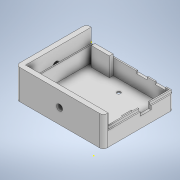
# Autodesk Inventor part: Shell 5 top
Saved by Autodesk Inventor 2022 (Build 260153000, 153)
## iProperties
Created: 2021-10-12
Part Number: Shell 5 top
Material: Generic
Document SubType Name: Modeling
Designer: Elisabeth
Density: 1 g/cm^3
Appearance: Default
Mass: 24.7843 g
Surface Area: 176.522 cm^2
Volume: 24.7843 cm^3
Author: Elisabeth
Autodesk Inventor part; units mm, degrees
ref_plane "YZ Plane" through (0, 0, 0) normal (1, 0, 0) x (0, 1, 0)
ref_plane "XZ Plane" through (0, 0, 0) normal (0, 1, 0) x (-1, 0, 0)
ref_plane "XY Plane" through (0, 0, 0) normal (0, 0, 1) x (1, 0, 0)
sketch "Sketch1" plane through (0, 0, 0) normal (0, 1, 0) x (-1, 0, 0)
  point P0 (0, 0)
sketch "Sketch2" plane through (0, 0, 0) normal (0, 1, 0) x (-1, 0, 0)
  line L0 (68, -12) -> (68, -66)
  line L1 (68, -66) -> (0, -66)
  line L2 (0, -66) -> (0, -12)
  line L3 (68, -12) -> (0, -12)
  point P0 (0, 0)
  dimension "d0" = 68
  dimension "d138" = 54
  constraints: 8 end point, 1 parallel, 1 perpendicular
  measures "d0" distance of L0.end L1.end
  measures "d138" distance between parallel lines of L3 L1
extrude "Extrusion1" add sketch "Sketch2" along normal blind 14
sketch "Sketch3" plane through (0, 14, 0) normal (0, 1, 0) x (1, 0, 0)
  point P0 (-68, 66)
sketch "Sketch4" plane through (0, 14, 0) normal (0, 1, 0) x (1, 0, 0)
  line L0 (0, 66) -> (-68, 66) projected
  line L1 (-30.4814, 66) -> (-28.4814, 66)
  line L2 (-28.4814, 66) -> (-28.4814, 64)
  line L3 (-68, 66) -> (-68, 12) projected
  line L4 (-68, 37.8423) -> (-68, 39.8423)
  line L5 (-68, 39.8423) -> (-66, 39.8423)
  line L6 (0, 38.8423) -> (0, 36.8423)
  line L7 (0, 36.8423) -> (-2, 36.8423)
  line L8 (-66, 64) -> (-2, 64)
  line L9 (-2, 64) -> (-2, 14)
  line L10 (-2, 14) -> (-66, 14)
  line L11 (-66, 14) -> (-66, 64)
  dimension "d5" = 2
  dimension "d6" = 2
  dimension "d7" = 2
  dimension "d11" = 2
  dimension "d75" = 2
  dimension "d132" = 50
  dimension "d133" = 64
  constraints: 20 end point, 4 perpendicular, 4 point on line, 2 parallel, 1 horizontal
  measures "d5" distance of L1.start L1.end
  measures "d6" distance of L1.end L2.end
  measures "d7" distance of L4.start L4.end
  measures "d11" distance of L6.start L6.end
  measures "d75" distance between parallel lines of L0 L8
  measures "d132" distance between parallel lines of L8 L10
  measures "d133" distance of L8.start L8.end
extrude "Extrusion2" cut sketch "Sketch4" against normal blind 13 contours L8 L9 L10 L11
sketch "Sketch7" plane through (0, 14, 0) normal (0, 1, 0) x (1, 0, 0)
  line L0 (-68, 66) -> (-67, 66)
  line L1 (-68, 66) -> (-6, 66)
  line L2 (-68, 65) -> (-68, 66)
  line L3 (0, 66) -> (-7, 66)
  line L4 (-67, 65) -> (-1, 65)
  line L5 (0, 66) -> (-68, 66) projected
  line L6 (-68, 66) -> (0, 66)
  line L7 (0, 12) -> (0, 66) projected
  line L8 (0, 12) -> (-1, 12)
  line L9 (-1, 66) -> (0, 66)
  line L10 (0, 66) -> (0, 12)
  line L11 (0, 12) -> (-1, 12)
  line L12 (-68, 12) -> (0, 12) projected
  line L13 (-1, 65) -> (-1, 12)
  line L14 (0, 12) -> (-1, 12)
  line L15 (-67, 65) -> (-67, 12)
  line L16 (-68, 66) -> (-68, 12) projected
  line L17 (-67, 12) -> (-68, 12)
  line L18 (-68, 12) -> (-68, 66)
  dimension "d76" = 1
  dimension "d139" = 1
  dimension "d140" = 1
  constraints: 30 end point, 6 horizontal, 3 collinear, 2 parallel, 2 perpendicular, 2 point on line
  measures "d76" distance between parallel lines of L1 L4
  measures "d139" distance between parallel lines of L7 L13
  measures "d140" distance between parallel lines of L16 L15
extrude "Extrusion3" cut sketch "Sketch7" against normal blind 2 contours L0 L1 L3 L7 L8 L13 L4 L15 L12 L16 L2
sketch "Sketch8" plane through (0, 14, 0) normal (0, 1, 0) x (1, 0, 0)
  line L0 (0, 12) -> (0, 13)
  line L1 (0, 13) -> (-68, 13)
  line L2 (0, 12) -> (-68, 12)
  line L3 (-68, 12) -> (-68, 13)
  line L4 (-67, 12) -> (-1, 12) projected
  point P0 (0, 0)
  point P1 (-70, 0)
  dimension "d46" = 68
  dimension "d141" = 1
  constraints: 8 end point, 1 horizontal, 1 perpendicular
  measures "d46" distance of L1.end L0.end
  measures "d141" distance of L0.start L0.end
extrude "Extrusion4" cut sketch "Sketch8" against normal blind 2
sketch "Sketch10" plane through (0, 1, 0) normal (0, 1, 0) x (1, 0, 0)
  line L0 (-31, 2) -> (-41, 2)
  line L1 (-63, 64) -> (-48, 64)
  line L2 (-48, 64) -> (-48, 61)
  line L3 (-48, 61) -> (-63, 61)
  line L4 (-63, 61) -> (-63, 64)
  line L5 (-22, 14) -> (-7, 14)
  line L6 (-7, 14) -> (-7, 17)
  line L7 (-7, 17) -> (-22, 17)
  line L8 (-22, 17) -> (-22, 14)
  line L9 (-66, 14) -> (-66, 64) projected
  line L10 (-2, 14) -> (-66, 14) projected
  line L11 (-66, 64) -> (-2, 64)
  line L12 (-2, 64) -> (-2, 14)
  line L13 (-2, 14) -> (-66, 14)
  line L14 (-66, 14) -> (-66, 64)
  point P0 (0, 0)
  point P1 (-21, 64)
  dimension "d57" = 15
  dimension "d58" = 3
  dimension "d61" = 15
  dimension "d79" = 3
  constraints: 26 end point, 6 parallel, 4 horizontal, 3 perpendicular, 1 other
  measures "d57" distance of L2.end L3.end
  measures "d58" distance of L1.end L2.end
  measures "d61" distance of L7.end L6.end
  measures "d79" distance between parallel lines of L7 L5
extrude "Extrusion5" add sketch "Sketch10" along normal blind 15.5 contours L1 L2 L3 L4 | L8 L7 L6 L5
sketch "Sketch11" plane through (0, 0, 0) normal (0, -1, 0) x (1, 0, 0)
  circle A0 centre (-12, -42.73) radius 4
  circle A1 centre (-33.5, -54.23) radius 1.5
  line L0 (0, 0) -> (0, -66) projected
  line L1 (0, -66) -> (-68, -66) projected
  line L2 (-2, -64) -> (-2, -14) projected
  dimension "d85" = 23.27
  dimension "d86" = 21.5
  dimension "d88" = 8
  dimension "d89" = 3
  dimension "d119" = 11.5
  dimension "d120" = 10
  constraints: 2 centre point
  measures "d85" distance from line of L1 A0.centre
  measures "d86" horizontal distance of A1.centre A0.centre
  measures "d88" diameter of A0
  measures "d89" diameter of A1
  measures "d119" vertical distance of A1.centre A0.centre
  measures "d120" distance from line of L2 A0.centre
extrude "Extrusion6" cut sketch "Sketch11" against normal blind 9
sketch "Sketch12" plane through (0, 0, 0) normal (0, -1, 0) x (1, 0, 0)
  line L0 (-68, -12) -> (-68, -66) projected
  line L1 (0, -12) -> (0, -8)
  line L2 (0, -8) -> (-68, -8)
  line L3 (-68, -12) -> (0, -12)
  line L4 (0, -12) -> (-68, -12) projected
  line L5 (-68, -66) -> (-68, -12) projected
  line L6 (-68, -66) -> (-72, -66)
  line L7 (-68, -12) -> (-68, -66)
  line L8 (-72, -66) -> (-72, -12)
  line L9 (-68, -8) -> (-72, -8)
  line L10 (-72, -8) -> (-72, -12.2471)
  point P0 (0, 0)
  point P1 (-70, 0)
  dimension "d81" = 4
  dimension "d144" = 0
  constraints: 16 end point, 2 horizontal, 2 point on line, 1 perpendicular, 1 vertical, 1 other
  measures "d81" distance of L1.end L1.start
  measures "d144" distance between parallel lines of L4 L3
extrude "Extrusion7" add sketch "Sketch12" against normal blind 24.5
sketch "Sketch15" plane through (0, 0, -66) normal (1, 0, 0) x (0, 0, -1)
  line L0 (-27.77, 14) -> (-18.77, 14)
  line L1 (-18.77, 14) -> (-18.77, 9)
  line L2 (-18.77, 9) -> (-27.77, 9)
  line L3 (-27.77, 9) -> (-27.77, 14)
  line L4 (-54, 0) -> (-54, 24.5) projected
  line L5 (0, 0) -> (0, 12) projected
  line L6 (0, 0) -> (-58, 0) projected
  line L7 (0, 12) -> (-54, 12) projected
  line L8 (-23.27, -7.8454) -> (-23.27, 0)
  line L9 (-23.27, 0) -> (-23.27, 12)
  line L10 (-53, 14) -> (-1, 14) projected
  point P0 (-66, 0)
  point P1 (-66, 14.75)
  point P2 (0, 16.75)
  point P3 (-1, 14)
  dimension "d108" = 9
  dimension "d109" = 5
  dimension "d111" = 27.77
  dimension "d174" = 0
  constraints: 12 end point, 2 parallel, 2 perpendicular, 2 point on line, 1 horizontal, 4 other
  measures "d108" distance of L1.end L2.end
  measures "d109" distance of L0.end L1.end
  measures "d111" distance between parallel lines of L5 L3
  measures "d174" vertical extent of L0
extrude "Extrusion9" cut sketch "Sketch15" against normal blind 10 contours L0 L1 L7 L3 | L7 L9 L2 L3 | L1 L2 L9 L7
fillet "Fillet7" radius 3 1 edges at (0, 6, -66)
fillet "Fillet9" radius 3 1 edges at (0, 12.25, -8)
sketch "Sketch17" plane through (-3, 0, -66) normal (0, 0, -1) x (-1, 0, 0)
  line L0 (2, 17) -> (10.5, 17)
  line L1 (10.5, 17) -> (10.5, 12)
  line L2 (10.5, 12) -> (2, 12)
  line L3 (2, 12) -> (2, 17)
  line L4 (17.1, 17) -> (25.6, 17)
  line L5 (25.6, 17) -> (25.6, 12)
  line L6 (25.6, 12) -> (17.1, 12)
  line L7 (17.1, 12) -> (17.1, 17)
  line L8 (66, 0) -> (66, 10.5) projected
  line L9 (-2, 14) -> (64, 14) projected
  line L10 (65, 12) -> (0, 12) projected
  line L11 (-3, 12) -> (-3, 0) projected
  point P0 (64, 10.5)
  point P1 (0, 12)
  dimension "d151" = 8.5
  dimension "d152" = 8.5
  dimension "d153" = 5
  dimension "d157" = 0
  dimension "d158" = 13.5
  dimension "d160" = 28.6
  constraints: 16 end point, 4 parallel, 2 horizontal, 2 perpendicular, 2 point on line, 1 other
  measures "d151" distance of L1.end L2.end
  measures "d152" distance of L5.end L6.end
  measures "d153" distance of L0.end L1.end
  measures "d157" vertical extent of L2
  measures "d158" distance between parallel lines of L11 L1
  measures "d160" distance between parallel lines of L5 L11
extrude "Extrusion11" cut sketch "Sketch17" against normal blind 10 contours L0 L1 L9 L3 | L9 L1 L2 L3 | L9 L5 L6 L7 | L7 L4 L5 L9
sketch "Sketch18" plane through (0, 1, 0) normal (0, 1, 0) x (1, 0, 0)
  circle A0 centre (-12, 42.73) radius 4 projected
  line L0 (-12, 38.73) -> (-8, 38.73)
  line L1 (-8, 38.73) -> (-8, 46.73)
  line L2 (-8, 46.73) -> (-16, 46.73)
  line L3 (-16, 46.73) -> (-16, 38.73)
  line L4 (-16, 38.73) -> (-12, 38.73)
  point P0 (0, 0)
  dimension "d169" = 4
  dimension "d170" = 8
  dimension "d171" = 8
  constraints: 10 end point, 4 perpendicular, 3 horizontal, 1 point on line, 1 vertical alignment, 1 other
  measures "d169" distance of L0.start L0.end
  measures "d170" distance of L0.end L1.end
  measures "d171" distance of L1.end L2.end
extrude "Extrusion12" cut sketch "Sketch18" against normal blind 1
sketch "Sketch19" plane through (-72, 0, -8) normal (0, 0, 1) x (1, 0, 0)
  line L0 (0, 24.5) -> (69, 24.5) projected
  line L1 (69, 0) -> (0, 0) projected
  line L2 (0, 24.5) -> (0, 0)
  line L3 (0, 0) -> (0, 24.5) projected
  line L4 (0, 12.25) -> (70, 12.25)
  line L5 (4, 12) -> (69, 12) projected
  line L6 (72, 12) -> (72, 0) projected
  line L7 (0, 0) -> (72, 0)
  line L8 (0, 4.6147) -> (36, 4.6147)
  line L9 (36, 4.6147) -> (36, 24.5)
  line L10 (72, 24.5) -> (4, 24.5) projected
  circle A0 centre (36, 12.25) radius 2.5
  dimension "d177" = 36
  dimension "d178" = 5
  constraints: 10 end point, 4 point on line, 2 parallel, 1 centre point, 1 horizontal, 1 midpoint, 1 perpendicular, 1 vertical
  measures "d177" distance of L8.start L8.end
  measures "d178" diameter of A0
extrude "Extrusion13" cut sketch "Sketch19" against normal blind 4 contours A0 L9 L4 | L4 L9 L5 A0 | A0 L4 L9 | L4 A0 L5 L9 | L5 L9 A0 | L9 L5 A0
sketch "Sketch20" plane through (-72, 0, -66) normal (-1, 0, 0) x (0, 0, 1)
  line L0 (0, 0) -> (0, 24.5) projected
  line L1 (0, 12.25) -> (58, 12.25)
  line L2 (58, 24.5) -> (58, 0) projected
  line L3 (3, 0) -> (55, 0) projected
  line L4 (29, 0) -> (29, 24.5)
  line L5 (54, 24.5) -> (0, 24.5) projected
  circle A0 centre (29, 12.25) radius 2.5
  point P0 (66, 0)
  dimension "d181" = 5
  constraints: 4 end point, 4 midpoint, 1 centre point, 1 point on line, 1 vertical
  measures "d181" diameter of A0
extrude "Extrusion14" cut sketch "Sketch20" against normal blind 4 contours A0 L4 L1 | L1 L4 A0 | L4 A0 L1 | L1 A0 L4
fillet "Fillet12" radius 3 1 edges at (-72, 12.25, -8)
fillet "Fillet13" radius 3 1 edges at (-72, 12.25, -66)
body "Solid1"
